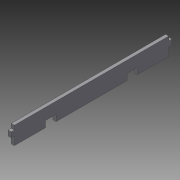
# Autodesk Inventor part: Electronics Chassis Wall
Saved by Autodesk Inventor 2015 (Build 190159000, 159)
## iProperties
Created: 2014-08-06
Part Number: Electronics Chassis Wall
Material: Generic
Document SubType Name: Modeling
Designer: STACKPOLE
Density: 1 g/cm^3
Appearance: Default
Author: STACKPOLE
Autodesk Inventor part; units mm, degrees
ref_plane "YZ Plane" through (0, 0, 0) normal (1, 0, 0) x (0, 1, 0)
ref_plane "XZ Plane" through (0, 0, 0) normal (0, 1, 0) x (-1, 0, 0)
ref_plane "XY Plane" through (0, 0, 0) normal (0, 0, 1) x (1, 0, 0)
sketch "Sketch1" plane through (0, 0, 0) normal (1, 0, 0) x (0, 1, 0)
  line L0 (0, 8) -> (-3, 8)
  line L1 (-3, 8) -> (-3, 13)
  line L2 (-3, 13) -> (0, 13)
  line L3 (0, 17) -> (0, 13)
  line L4 (0, 8) -> (0, 0)
  line L5 (148, 13) -> (151, 13)
  line L6 (151, 13) -> (151, 8)
  line L7 (151, 8) -> (148, 8)
  line L8 (148, 0) -> (148, 8)
  line L9 (148, 13) -> (148, 17)
  line L10 (30, 0) -> (30, 6)
  line L11 (30, 6) -> (40, 6)
  line L12 (40, 6) -> (40, 0)
  line L13 (108, 0) -> (108, 6)
  line L14 (108, 6) -> (118, 6)
  line L15 (118, 6) -> (118, 0)
  line L16 (40, 0) -> (108, 0)
  line L17 (148, 17) -> (0, 17)
  line L18 (30, 0) -> (0, 0)
  line L19 (118, 0) -> (148, 0)
  dimension "d1" = 148
  dimension "d2" = 5
  dimension "d3" = 3
  dimension "d7" = 10
  dimension "d9" = 30
  dimension "d31" = 6
  dimension "d38" = 17
  dimension "d39" = 8
  dimension "d40" = 2
  constraints: 40 end point, 15 perpendicular, 7 parallel, 5 equal length, 3 horizontal, 2 collinear, 2 vertical alignment, 1 coincident, 1 horizontal alignment
  measures "d1" distance of point (0, 0) L8.start
  measures "d2" distance of L0.end L1.end
  measures "d3" distance of L0.start L0.end
  measures "d7" distance of L10.end L11.end
  measures "d9" distance between parallel lines of L4 L10
  measures "d31" distance between parallel lines of L16 L11
  measures "d38" distance between parallel lines of L18 L17
  measures "d39" distance between parallel lines of L18 L0
  measures "d40" distance between parallel lines of L11 L0
extrude "Extrusion2" add sketch "Sketch1" along normal blind 3
body "Solid2"
